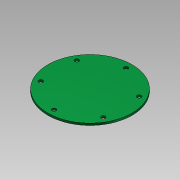
# Autodesk Inventor part: capsule.electronics.board
Saved by Autodesk Inventor 2011 (Build 150239000, 239)
## iProperties
Created: 2011-01-27
Part Number: capsule.electronics.board
Document SubType Name: Modeling
Designer: Casey
Density: 1 g/cm^3
Author: Casey
Autodesk Inventor part; units mm, degrees
ref_plane "YZ Plane" through (0, 0, 0) normal (1, 0, 0) x (0, 1, 0)
ref_plane "XZ Plane" through (0, 0, 0) normal (0, 1, 0) x (-1, 0, 0)
ref_plane "XY Plane" through (0, 0, 0) normal (0, 0, 1) x (1, 0, 0)
sketch "Sketch1" plane through (0, 0, 0) normal (0, 0, 1) x (1, 0, 0)
  circle A0 centre (0, 0) radius 35
  point P0 (0, 30)
  point P1 (-25.9808, 15)
  point P2 (-25.9808, -15)
  point P3 (0, -30)
  point P4 (25.9808, -15)
  point P5 (25.9808, 15)
  dimension "d0" = 30
  dimension "d1" = 70
  dimension "d13" = 360
  constraints: 1 centre point, 1 coincident, 7 other
  measures "d0" distance of A0.centre point (0, 30)
  measures "d1" diameter of A0
extrude "Extrusion1" add sketch "Sketch1" along normal blind 1.66
hole "Hole1" at (0, 30, 0) at (25.9808, 15, 0) at (0, -30, 0) at (-25.9808, -15, 0) at (-25.9808, 15, 0) at (25.9808, -15, 0) direction (0, 0, 1) diameter 3.4 depth 8 tip angle 118 clearance for "Flat Head Machine Screw" size "M3" standard "Ansi Metric M Profile"
body "Solid1"
